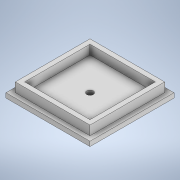
# Autodesk Inventor part: BlackBoxTopFall2019
Saved by Autodesk Inventor 2020 (Build 240168000, 168)
## iProperties
Created: 2019-09-20
Part Number: BlackBoxTopFall2019
Material: Generic
Document SubType Name: Modeling
Designer: hwatsky
Density: 1 g/cm^3
Appearance: Default
Author: hwatsky
Autodesk Inventor part; units mm, degrees
ref_plane "YZ Plane" through (0, 0, 0) normal (1, 0, 0) x (0, 1, 0)
ref_plane "XZ Plane" through (0, 0, 0) normal (0, 1, 0) x (-1, 0, 0)
ref_plane "XY Plane" through (0, 0, 0) normal (0, 0, 1) x (1, 0, 0)
sketch "Sketch1" plane through (0, 0, 0) normal (0, 1, 0) x (-1, 0, 0)
  line L0 (0, 0) -> (90, 0)
  line L1 (90, 0) -> (90, -90)
  line L2 (90, -90) -> (0, -90)
  line L3 (0, -90) -> (0, 0)
  dimension "d0" = 90
  dimension "d1" = 90
  constraints: 8 end point, 2 parallel, 1 horizontal, 1 perpendicular
  measures "d0" distance of L0.end L1.end
  measures "d1" distance of L1.end L2.end
extrude "Extrusion1" add sketch "Sketch1" along normal blind 5
sketch "Sketch2" plane through (0, 5, 0) normal (0, 1, 0) x (1, 0, 0)
  line L0 (-5, 5) -> (-85, 5)
  line L1 (-85, 5) -> (-85, 85)
  line L2 (-85, 85) -> (-5, 85)
  line L3 (-5, 85) -> (-5, 5)
  line L4 (0, 0) -> (0, 90) projected
  line L5 (-90, 0) -> (0, 0) projected
  line L6 (-10, 10) -> (-80, 10)
  line L7 (-80, 10) -> (-80, 80)
  line L8 (-80, 80) -> (-10, 80)
  line L9 (-10, 80) -> (-10, 10)
  dimension "d4" = 5
  dimension "d5" = 5
  dimension "d6" = 80
  dimension "d7" = 80
  dimension "d8" = 5
  dimension "d9" = 5
  dimension "d10" = 70
  dimension "d11" = 70
  constraints: 16 end point, 4 parallel, 2 horizontal, 2 perpendicular
  measures "d4" distance between parallel lines of L4 L3
  measures "d5" distance between parallel lines of L5 L0
  measures "d6" distance of L1.end L2.end
  measures "d7" distance of L2.end L0.start
  measures "d8" distance between parallel lines of L3 L9
  measures "d9" distance between parallel lines of L0 L6
  measures "d10" distance of L8.end L6.start
  measures "d11" distance of L6.start L6.end
extrude "Extrusion2" add sketch "Sketch2" along normal blind 10
sketch "Sketch3" plane through (0, 5, 0) normal (0, 1, 0) x (1, 0, 0)
  circle A0 centre (-45, 45) radius 3.5
  line L0 (0, 0) -> (0, 90) projected
  line L1 (0, 90) -> (-90, 90) projected
  dimension "d14" = 45
  dimension "d15" = 45
  dimension "d16" = 7
  constraints: 1 centre point
  measures "d14" distance from line of L0 A0.centre
  measures "d15" distance from line of L1 A0.centre
  measures "d16" diameter of A0
extrude "Extrusion3" cut sketch "Sketch3" against normal blind 10
body "Solid1"
